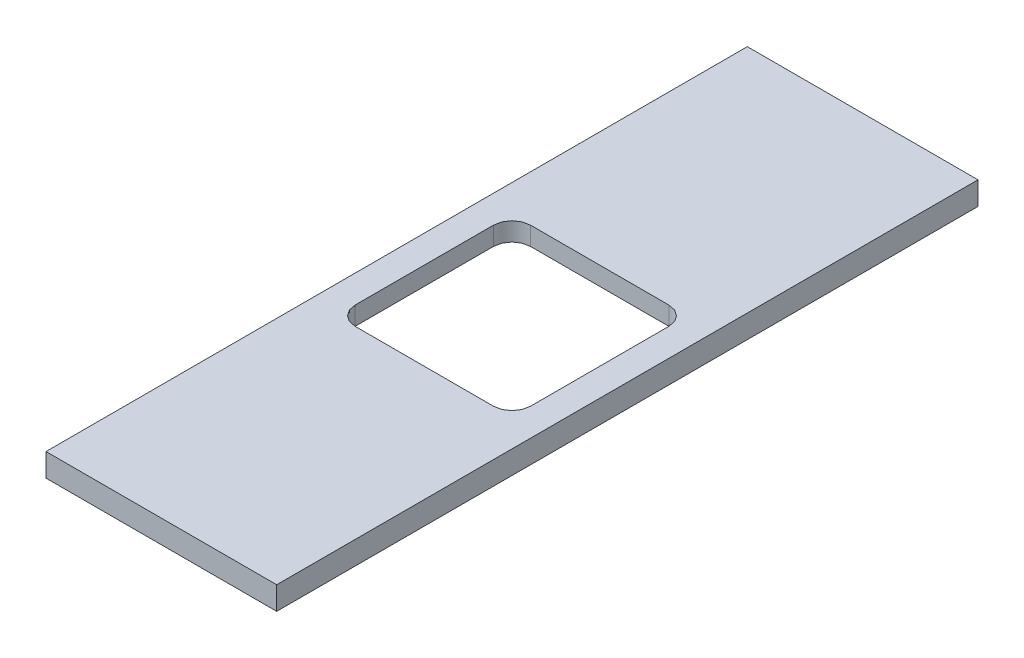
# Autodesk Inventor part: scope coverslip holder lowpro
Saved by Autodesk Inventor 2022 (Build 260153000, 153)
## iProperties
Created: 2019-09-11
Part Number: scope coverslip holder lowpro
Material: Generic
Document SubType Name: Modeling
Designer: Eamon
Density: 1 g/cm^3
Appearance: Default
Author: Eamon
Autodesk Inventor part; units mm, degrees
ref_plane "YZ Plane" through (0, 0, 0) normal (1, 0, 0) x (0, 1, 0)
ref_plane "XZ Plane" through (0, 0, 0) normal (0, 1, 0) x (-1, 0, 0)
ref_plane "XY Plane" through (0, 0, 0) normal (0, 0, 1) x (1, 0, 0)
sketch "Sketch1" plane through (0, 0, 0) normal (0, 1, 0) x (-1, 0, 0)
  line L0 (0, 0) -> (25, 0)
  line L1 (25, 0) -> (25, -76)
  line L2 (25, -76) -> (0, -76)
  line L3 (0, -76) -> (0, 0)
  dimension "d0" = 76
  dimension "d1" = 25
  constraints: 8 end point, 2 parallel, 1 horizontal, 1 perpendicular
  measures "d0" distance of L2.end L0.start
  measures "d1" distance of L0.start L0.end
extrude "Extrusion1" add sketch "Sketch1" along normal blind 2.5
ref_plane "Work Plane2" through (0, 5.5, 0) normal (0, 1, 0) x (1, 0, 0)
sketch "Sketch3" plane through (0, 5.5, 0) normal (0, 1, 0) x (1, 0, 0)
  line L0 (0, 0) -> (-25, 0) construction
  line L1 (-12.5, 0) -> (-12.5, 76) construction
  line L2 (-25, 76) -> (0, 76) construction
  line L3 (-25, 71) -> (-25, 5) construction
  line L4 (-25, 38) -> (-0.4405, 38) construction
  line L5 (-20, 28.5) -> (-5, 28.5)
  line L6 (-3, 30.5) -> (-3, 45.5)
  line L7 (-5, 47.5) -> (-20, 47.5)
  line L8 (-22, 45.5) -> (-22, 30.5)
  line L9 (-22, 28.5) -> (-3, 47.5) construction
  line L10 (-3, 28.5) -> (-22, 47.5) construction
  arc A0 (-20, 47.5) -> (-22, 45.5) centre (-20, 45.5) ccw
  arc A1 (-3, 45.5) -> (-5, 47.5) centre (-5, 45.5) ccw
  arc A2 (-5, 28.5) -> (-3, 30.5) centre (-5, 30.5) ccw
  arc A3 (-22, 30.5) -> (-20, 28.5) centre (-20, 30.5) ccw
  point P0 (-12.5, 38)
  dimension "d8" = 19
  dimension "d9" = 2
  dimension "d10" = 2
  dimension "d11" = 2
  dimension "d12" = 2
  constraints: 16 end point, 9 point on line, 8 point on circle, 8 tangent, 6 midpoint, 4 centre point, 2 parallel, 2 perpendicular, 1 horizontal, 1 vertical
  measures "d8" distance of L9.end L10.end
  measures "d9" radius of A0
  measures "d10" radius of A1
  measures "d11" radius of A2
  measures "d12" radius of A3
extrude "Extrusion3" cut sketch "Sketch3" against normal blind 6
sketch "Sketch4" plane through (0, 0, 0) normal (0, -1, 0) x (1, 0, 0)
  line L0 (0, -76) -> (0, 0) construction
  line L1 (0, -38) -> (-25, -38) construction
  line L2 (-25, -71) -> (-25, -5) construction
  line L3 (0, 0) -> (-25, 0) construction
  line L4 (-12.5, 0) -> (-12.5, -76) construction
  line L5 (-25, -76) -> (0, -76) construction
  line L6 (-19.875, -49.375) -> (-5.125, -49.375)
  line L7 (-1.125, -49.375) -> (-1.125, -26.625)
  line L8 (-5.125, -26.625) -> (-19.875, -26.625)
  line L9 (-23.875, -26.625) -> (-23.875, -49.375)
  line L10 (-23.875, -49.375) -> (-1.125, -26.625) construction
  line L11 (-1.125, -49.375) -> (-23.875, -26.625) construction
  arc A0 (-1.125, -26.625) -> (-5.125, -26.625) centre (-3.125, -26.625) ccw
  arc A1 (-19.875, -26.625) -> (-23.875, -26.625) centre (-21.875, -26.625) ccw
  arc A2 (-23.875, -49.375) -> (-19.875, -49.375) centre (-21.875, -49.375) ccw
  arc A3 (-5.125, -49.375) -> (-1.125, -49.375) centre (-3.125, -49.375) ccw
  point P0 (-12.5, -38)
  dimension "d15" = 22.75
  dimension "d16" = 4
  dimension "d17" = 22.75
  constraints: 16 end point, 8 point on circle, 7 midpoint, 4 centre point, 4 point on line, 4 vertical alignment, 3 equal radius, 3 horizontal alignment, 2 parallel, 1 horizontal, 1 perpendicular, 1 tangent
  measures "d15" distance of L7.end L9.start
  measures "d16" diameter of A0
  measures "d17" distance of L7.start L7.end
extrude "Extrusion4" cut sketch "Sketch4" against normal blind 0.5
sketch "Sketch5" plane through (0, 0, 0) normal (0, -1, 0) x (1, 0, 0)
  circle A0 centre (-12.5, -19.3349) radius 2.5305
  circle A1 centre (-12.5, -56) radius 2.6164
  line L0 (0, -76) -> (0, 0) projected
  line L1 (-25, -76) -> (0, -76) projected
  dimension "d20" = 12.5
  dimension "d21" = 20
  constraints: 2 centre point, 1 vertical alignment
  measures "d20" distance from line of L0 A1.centre
  measures "d21" distance from line of L1 A1.centre
body "Solid1"
